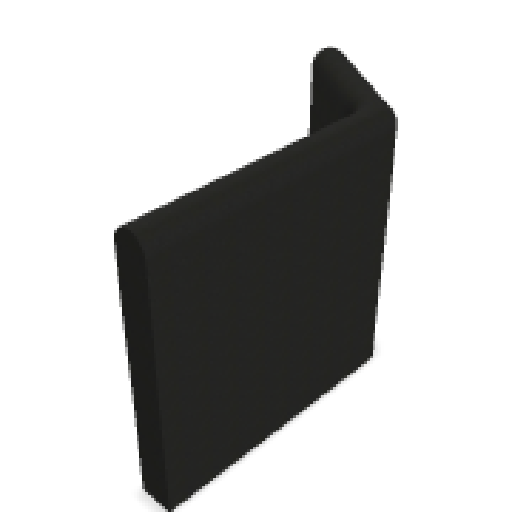
# Autodesk Inventor part: wall
Saved by Autodesk Inventor 2023 (Build 270158000, 158)
## iProperties
Created: 2022-08-08
Part Number: wall
Material: Generic
Document SubType Name: Modeling
Designer: Derm
Density: 1 g/cm^3
Appearance: Smooth - Beige
Author: Derm
Autodesk Inventor part; units mm, degrees
ref_plane "YZ Plane" through (0, 0, 0) normal (1, 0, 0) x (0, 1, 0)
ref_plane "XZ Plane" through (0, 0, 0) normal (0, 1, 0) x (-1, 0, 0)
ref_plane "XY Plane" through (0, 0, 0) normal (0, 0, 1) x (1, 0, 0)
sketch "Sketch1" plane through (0, 0, 0) normal (0, 0, 1) x (1, 0, 0)
  line L0 (0, 0) -> (500, 0)
  line L1 (500, 0) -> (500, 4000)
  line L2 (500, 4000) -> (0, 4000)
  line L3 (0, 4000) -> (0, 0)
  point P0 (250, 0)
  dimension "d0" = 500
  dimension "d1" = 4000
  constraints: 8 end point, 2 parallel, 1 horizontal, 1 midpoint, 1 perpendicular
  measures "d0" distance between parallel lines of L1 L3
  measures "d1" distance from line of point (250, 0) L2
extrude "Extrusion1" add sketch "Sketch1" along normal mid plane 3000
sketch "Sketch2" plane through (0, 4000, 1500) normal (0, 1, 0) x (1, 0, 0)
  line L0 (0, 3000) -> (0, 0) projected
  line L1 (500, 0) -> (0, 0) projected
  line L2 (500, 3000) -> (500, 0) projected
  line L3 (0, 3000) -> (500, 3000) projected
  line L4 (500, 3000) -> (-1473.7429, 4196.0586)
  line L5 (0, 2718.352) -> (-1732.8702, 3768.4454)
  line L6 (-1473.7429, 4196.0586) -> (-1732.8702, 3768.4454)
  point P0 (0, 1500)
  dimension "d18" = 500
  constraints: 6 end point, 1 parallel, 1 perpendicular, 1 point on line
  measures "d18" distance between parallel lines of L4 L5
extrude "Extrusion4" add sketch "Sketch2" against normal up to surface (4000 mm away) contours L0 L5 L6 L4 L3
fillet "Fillet2" radius 304.8 2 edges at (500, 2000, -1500) (0, 2000, -1218.352)
fillet "Fillet3" [suppressed]
fillet "Fillet4" [suppressed]
sketch "Sketch4" plane through (0, 0, 1500) normal (0, 0, 1) x (1, 0, 0)
  line L0 (0, 4000) -> (0, 0) projected
  line L1 (0, 0) -> (500, 0) projected
  line L2 (500, 0) -> (500, 4000) projected
  line L3 (500, 4000) -> (0, 4000) projected
extrude "Extrusion5" add sketch "Sketch4" along normal blind 1000
body "Solid1"
